Autodesk Inventor part; units mm, degrees
(part 6 of 6)
  arc A2821 (-284.9898, 50) -> (-285.1385, 49.8696) centre (-284.9898, 49.85) ccw
  line L381 (-284.9898, 50) -> (-284.4705, 50)
  arc A2822 (-284.3218, 49.8696) -> (-284.4705, 50) centre (-284.4705, 49.85) ccw
  arc A2823 (-284.3218, 49.8696) -> (-284.2292, 49.5618) centre (-283.3304, 50) ccw
  arc A2824 (-284.2292, 49.5618) -> (-283.7302, 49.25) centre (-283.7304, 49.805) ccw
  arc A2825 (-283.7302, 49.25) -> (-283.2311, 49.5618) centre (-283.73, 49.805) ccw
  arc A2826 (-283.2311, 49.5618) -> (-283.1385, 49.8696) centre (-284.13, 50) ccw
  arc A2827 (-282.9898, 50) -> (-283.1385, 49.8696) centre (-282.9898, 49.85) ccw
  line L382 (-282.9898, 50) -> (-282.4705, 50)
  arc A2828 (-282.3218, 49.8696) -> (-282.4705, 50) centre (-282.4705, 49.85) ccw
  arc A2829 (-282.3218, 49.8696) -> (-282.2292, 49.5618) centre (-281.3304, 50) ccw
  arc A2830 (-282.2292, 49.5618) -> (-281.7302, 49.25) centre (-281.7304, 49.805) ccw
  arc A2831 (-281.7302, 49.25) -> (-281.2311, 49.5618) centre (-281.73, 49.805) ccw
  arc A2832 (-281.2311, 49.5618) -> (-281.1385, 49.8696) centre (-282.13, 50) ccw
  arc A2833 (-280.9898, 50) -> (-281.1385, 49.8696) centre (-280.9898, 49.85) ccw
  line L383 (-280.9898, 50) -> (-280.4705, 50)
  arc A2834 (-280.3218, 49.8696) -> (-280.4705, 50) centre (-280.4705, 49.85) ccw
  arc A2835 (-280.3218, 49.8696) -> (-280.2292, 49.5618) centre (-279.3304, 50) ccw
  arc A2836 (-280.2292, 49.5618) -> (-279.7302, 49.25) centre (-279.7304, 49.805) ccw
  arc A2837 (-279.7302, 49.25) -> (-279.2311, 49.5618) centre (-279.73, 49.805) ccw
  arc A2838 (-279.2311, 49.5618) -> (-279.1385, 49.8696) centre (-280.13, 50) ccw
  arc A2839 (-278.9898, 50) -> (-279.1385, 49.8696) centre (-278.9898, 49.85) ccw
  line L384 (-278.9898, 50) -> (-278.4705, 50)
  arc A2840 (-278.3218, 49.8696) -> (-278.4705, 50) centre (-278.4705, 49.85) ccw
  arc A2841 (-278.3218, 49.8696) -> (-278.2292, 49.5618) centre (-277.3304, 50) ccw
  arc A2842 (-278.2292, 49.5618) -> (-277.7302, 49.25) centre (-277.7304, 49.805) ccw
  arc A2843 (-277.7302, 49.25) -> (-277.2311, 49.5618) centre (-277.73, 49.805) ccw
  arc A2844 (-277.2311, 49.5618) -> (-277.1385, 49.8696) centre (-278.13, 50) ccw
  arc A2845 (-276.9898, 50) -> (-277.1385, 49.8696) centre (-276.9898, 49.85) ccw
  line L385 (-276.9898, 50) -> (-276.4705, 50)
  arc A2846 (-276.3218, 49.8696) -> (-276.4705, 50) centre (-276.4705, 49.85) ccw
  arc A2847 (-276.3218, 49.8696) -> (-276.2292, 49.5618) centre (-275.3304, 50) ccw
  arc A2848 (-276.2292, 49.5618) -> (-275.7302, 49.25) centre (-275.7304, 49.805) ccw
  arc A2849 (-275.7302, 49.25) -> (-275.2311, 49.5618) centre (-275.73, 49.805) ccw
  arc A2850 (-275.2311, 49.5618) -> (-275.1385, 49.8696) centre (-276.13, 50) ccw
  arc A2851 (-274.9898, 50) -> (-275.1385, 49.8696) centre (-274.9898, 49.85) ccw
  line L386 (-274.9898, 50) -> (-274.4705, 50)
  arc A2852 (-274.3218, 49.8696) -> (-274.4705, 50) centre (-274.4705, 49.85) ccw
  arc A2853 (-274.3218, 49.8696) -> (-274.2292, 49.5618) centre (-273.3304, 50) ccw
  arc A2854 (-274.2292, 49.5618) -> (-273.7302, 49.25) centre (-273.7304, 49.805) ccw
  arc A2855 (-273.7302, 49.25) -> (-273.2311, 49.5618) centre (-273.73, 49.805) ccw
  arc A2856 (-273.2311, 49.5618) -> (-273.1385, 49.8696) centre (-274.13, 50) ccw
  arc A2857 (-272.9898, 50) -> (-273.1385, 49.8696) centre (-272.9898, 49.85) ccw
  line L387 (-272.9898, 50) -> (-272.4705, 50)
  arc A2858 (-272.3218, 49.8696) -> (-272.4705, 50) centre (-272.4705, 49.85) ccw
  arc A2859 (-272.3218, 49.8696) -> (-272.2292, 49.5618) centre (-271.3304, 50) ccw
  arc A2860 (-272.2292, 49.5618) -> (-271.7302, 49.25) centre (-271.7304, 49.805) ccw
  arc A2861 (-271.7302, 49.25) -> (-271.2311, 49.5618) centre (-271.73, 49.805) ccw
  arc A2862 (-271.2311, 49.5618) -> (-271.1385, 49.8696) centre (-272.13, 50) ccw
  arc A2863 (-270.9898, 50) -> (-271.1385, 49.8696) centre (-270.9898, 49.85) ccw
  line L388 (-270.9898, 50) -> (-270.4705, 50)
  arc A2864 (-270.3218, 49.8696) -> (-270.4705, 50) centre (-270.4705, 49.85) ccw
  arc A2865 (-270.3218, 49.8696) -> (-270.2292, 49.5618) centre (-269.3304, 50) ccw
  arc A2866 (-270.2292, 49.5618) -> (-269.7302, 49.25) centre (-269.7304, 49.805) ccw
  arc A2867 (-269.7302, 49.25) -> (-269.2311, 49.5618) centre (-269.73, 49.805) ccw
  arc A2868 (-269.2311, 49.5618) -> (-269.1385, 49.8696) centre (-270.13, 50) ccw
  arc A2869 (-268.9898, 50) -> (-269.1385, 49.8696) centre (-268.9898, 49.85) ccw
  line L389 (-268.9898, 50) -> (-268.4705, 50)
  arc A2870 (-268.3218, 49.8696) -> (-268.4705, 50) centre (-268.4705, 49.85) ccw
  arc A2871 (-268.3218, 49.8696) -> (-268.2292, 49.5618) centre (-267.3304, 50) ccw
  arc A2872 (-268.2292, 49.5618) -> (-267.7302, 49.25) centre (-267.7304, 49.805) ccw
  arc A2873 (-267.7302, 49.25) -> (-267.2311, 49.5618) centre (-267.73, 49.805) ccw
  arc A2874 (-267.2311, 49.5618) -> (-267.1385, 49.8696) centre (-268.13, 50) ccw
  arc A2875 (-266.9898, 50) -> (-267.1385, 49.8696) centre (-266.9898, 49.85) ccw
  line L390 (-266.9898, 50) -> (-266.4705, 50)
  arc A2876 (-266.3218, 49.8696) -> (-266.4705, 50) centre (-266.4705, 49.85) ccw
  arc A2877 (-266.3218, 49.8696) -> (-266.2292, 49.5618) centre (-265.3304, 50) ccw
  arc A2878 (-266.2292, 49.5618) -> (-265.7302, 49.25) centre (-265.7304, 49.805) ccw
  arc A2879 (-265.7302, 49.25) -> (-265.2311, 49.5618) centre (-265.73, 49.805) ccw
  arc A2880 (-265.2311, 49.5618) -> (-265.1385, 49.8696) centre (-266.13, 50) ccw
  arc A2881 (-264.9898, 50) -> (-265.1385, 49.8696) centre (-264.9898, 49.85) ccw
  line L391 (-264.9898, 50) -> (-264.4705, 50)
  arc A2882 (-264.3218, 49.8696) -> (-264.4705, 50) centre (-264.4705, 49.85) ccw
  arc A2883 (-264.3218, 49.8696) -> (-264.2292, 49.5618) centre (-263.3304, 50) ccw
  arc A2884 (-264.2292, 49.5618) -> (-263.7302, 49.25) centre (-263.7304, 49.805) ccw
  arc A2885 (-263.7302, 49.25) -> (-263.2311, 49.5618) centre (-263.73, 49.805) ccw
  arc A2886 (-263.2311, 49.5618) -> (-263.1385, 49.8696) centre (-264.13, 50) ccw
  arc A2887 (-262.9898, 50) -> (-263.1385, 49.8696) centre (-262.9898, 49.85) ccw
  line L392 (-262.9898, 50) -> (-262.4705, 50)
  arc A2888 (-262.3218, 49.8696) -> (-262.4705, 50) centre (-262.4705, 49.85) ccw
  arc A2889 (-262.3218, 49.8696) -> (-262.2292, 49.5618) centre (-261.3304, 50) ccw
  arc A2890 (-262.2292, 49.5618) -> (-261.7302, 49.25) centre (-261.7304, 49.805) ccw
  arc A2891 (-261.7302, 49.25) -> (-261.2311, 49.5618) centre (-261.73, 49.805) ccw
  arc A2892 (-261.2311, 49.5618) -> (-261.1385, 49.8696) centre (-262.13, 50) ccw
  arc A2893 (-260.9898, 50) -> (-261.1385, 49.8696) centre (-260.9898, 49.85) ccw
  line L393 (-260.9898, 50) -> (-260.4705, 50)
  arc A2894 (-260.3218, 49.8696) -> (-260.4705, 50) centre (-260.4705, 49.85) ccw
  arc A2895 (-260.3218, 49.8696) -> (-260.2292, 49.5618) centre (-259.3304, 50) ccw
  arc A2896 (-260.2292, 49.5618) -> (-259.7302, 49.25) centre (-259.7304, 49.805) ccw
  arc A2897 (-259.7302, 49.25) -> (-259.2311, 49.5618) centre (-259.73, 49.805) ccw
  arc A2898 (-259.2311, 49.5618) -> (-259.1385, 49.8696) centre (-260.13, 50) ccw
  arc A2899 (-258.9898, 50) -> (-259.1385, 49.8696) centre (-258.9898, 49.85) ccw
  line L394 (-258.9898, 50) -> (-258.4705, 50)
  arc A2900 (-258.3218, 49.8696) -> (-258.4705, 50) centre (-258.4705, 49.85) ccw
  arc A2901 (-258.3218, 49.8696) -> (-258.2292, 49.5618) centre (-257.3304, 50) ccw
  arc A2902 (-258.2292, 49.5618) -> (-257.7302, 49.25) centre (-257.7304, 49.805) ccw
  arc A2903 (-257.7302, 49.25) -> (-257.2311, 49.5618) centre (-257.73, 49.805) ccw
  arc A2904 (-257.2311, 49.5618) -> (-257.1385, 49.8696) centre (-258.13, 50) ccw
  arc A2905 (-256.9898, 50) -> (-257.1385, 49.8696) centre (-256.9898, 49.85) ccw
  line L395 (-256.9898, 50) -> (-256.4705, 50)
  arc A2906 (-256.3218, 49.8696) -> (-256.4705, 50) centre (-256.4705, 49.85) ccw
  arc A2907 (-256.3218, 49.8696) -> (-256.2292, 49.5618) centre (-255.3304, 50) ccw
  arc A2908 (-256.2292, 49.5618) -> (-255.7302, 49.25) centre (-255.7304, 49.805) ccw
  arc A2909 (-255.7302, 49.25) -> (-255.2311, 49.5618) centre (-255.73, 49.805) ccw
  arc A2910 (-255.2311, 49.5618) -> (-255.1385, 49.8696) centre (-256.13, 50) ccw
  arc A2911 (-254.9898, 50) -> (-255.1385, 49.8696) centre (-254.9898, 49.85) ccw
  line L396 (-254.9898, 50) -> (-254.4705, 50)
  arc A2912 (-254.3218, 49.8696) -> (-254.4705, 50) centre (-254.4705, 49.85) ccw
  arc A2913 (-254.3218, 49.8696) -> (-254.2292, 49.5618) centre (-253.3304, 50) ccw
  arc A2914 (-254.2292, 49.5618) -> (-253.7302, 49.25) centre (-253.7304, 49.805) ccw
  arc A2915 (-253.7302, 49.25) -> (-253.2311, 49.5618) centre (-253.73, 49.805) ccw
  arc A2916 (-253.2311, 49.5618) -> (-253.1385, 49.8696) centre (-254.13, 50) ccw
  arc A2917 (-252.9898, 50) -> (-253.1385, 49.8696) centre (-252.9898, 49.85) ccw
  line L397 (-252.9898, 50) -> (-252.4705, 50)
  arc A2918 (-252.3218, 49.8696) -> (-252.4705, 50) centre (-252.4705, 49.85) ccw
  arc A2919 (-252.3218, 49.8696) -> (-252.2292, 49.5618) centre (-251.3304, 50) ccw
  arc A2920 (-252.2292, 49.5618) -> (-251.7302, 49.25) centre (-251.7304, 49.805) ccw
  arc A2921 (-251.7302, 49.25) -> (-251.2311, 49.5618) centre (-251.73, 49.805) ccw
  arc A2922 (-251.2311, 49.5618) -> (-251.1385, 49.8696) centre (-252.13, 50) ccw
  arc A2923 (-250.9898, 50) -> (-251.1385, 49.8696) centre (-250.9898, 49.85) ccw
  line L398 (-250.9898, 50) -> (-250.4705, 50)
  arc A2924 (-250.3218, 49.8696) -> (-250.4705, 50) centre (-250.4705, 49.85) ccw
  arc A2925 (-250.3218, 49.8696) -> (-250.2292, 49.5618) centre (-249.3304, 50) ccw
  arc A2926 (-250.2292, 49.5618) -> (-249.7302, 49.25) centre (-249.7304, 49.805) ccw
  arc A2927 (-249.7302, 49.25) -> (-249.2311, 49.5618) centre (-249.73, 49.805) ccw
  arc A2928 (-249.2311, 49.5618) -> (-249.1385, 49.8696) centre (-250.13, 50) ccw
  arc A2929 (-248.9898, 50) -> (-249.1385, 49.8696) centre (-248.9898, 49.85) ccw
  line L399 (-248.9898, 50) -> (-248.4705, 50)
  arc A2930 (-248.3218, 49.8696) -> (-248.4705, 50) centre (-248.4705, 49.85) ccw
  arc A2931 (-248.3218, 49.8696) -> (-248.2292, 49.5618) centre (-247.3304, 50) ccw
  arc A2932 (-248.2292, 49.5618) -> (-247.7302, 49.25) centre (-247.7304, 49.805) ccw
  arc A2933 (-247.7302, 49.25) -> (-247.2311, 49.5618) centre (-247.73, 49.805) ccw
  arc A2934 (-247.2311, 49.5618) -> (-247.1385, 49.8696) centre (-248.13, 50) ccw
  arc A2935 (-246.9898, 50) -> (-247.1385, 49.8696) centre (-246.9898, 49.85) ccw
  line L400 (-246.9898, 50) -> (-246.4705, 50)
  arc A2936 (-246.3218, 49.8696) -> (-246.4705, 50) centre (-246.4705, 49.85) ccw
  arc A2937 (-246.3218, 49.8696) -> (-246.2292, 49.5618) centre (-245.3304, 50) ccw
  arc A2938 (-246.2292, 49.5618) -> (-245.7302, 49.25) centre (-245.7304, 49.805) ccw
  arc A2939 (-245.7302, 49.25) -> (-245.2311, 49.5618) centre (-245.73, 49.805) ccw
  arc A2940 (-245.2311, 49.5618) -> (-245.1385, 49.8696) centre (-246.13, 50) ccw
  arc A2941 (-244.9898, 50) -> (-245.1385, 49.8696) centre (-244.9898, 49.85) ccw
  line L401 (-244.9898, 50) -> (-244.4705, 50)
  arc A2942 (-244.3218, 49.8696) -> (-244.4705, 50) centre (-244.4705, 49.85) ccw
  arc A2943 (-244.3218, 49.8696) -> (-244.2292, 49.5618) centre (-243.3304, 50) ccw
  arc A2944 (-244.2292, 49.5618) -> (-243.7302, 49.25) centre (-243.7304, 49.805) ccw
  arc A2945 (-243.7302, 49.25) -> (-243.2311, 49.5618) centre (-243.73, 49.805) ccw
  arc A2946 (-243.2311, 49.5618) -> (-243.1385, 49.8696) centre (-244.13, 50) ccw
  arc A2947 (-242.9898, 50) -> (-243.1385, 49.8696) centre (-242.9898, 49.85) ccw
  line L402 (-242.9898, 50) -> (-242.4705, 50)
  arc A2948 (-242.3218, 49.8696) -> (-242.4705, 50) centre (-242.4705, 49.85) ccw
  arc A2949 (-242.3218, 49.8696) -> (-242.2292, 49.5618) centre (-241.3304, 50) ccw
  arc A2950 (-242.2292, 49.5618) -> (-241.7302, 49.25) centre (-241.7304, 49.805) ccw
  arc A2951 (-241.7302, 49.25) -> (-241.2311, 49.5618) centre (-241.73, 49.805) ccw
  arc A2952 (-241.2311, 49.5618) -> (-241.1385, 49.8696) centre (-242.13, 50) ccw
  arc A2953 (-240.9898, 50) -> (-241.1385, 49.8696) centre (-240.9898, 49.85) ccw
  line L403 (-240.9898, 50) -> (-240.4705, 50)
  arc A2954 (-240.3218, 49.8696) -> (-240.4705, 50) centre (-240.4705, 49.85) ccw
  arc A2955 (-240.3218, 49.8696) -> (-240.2292, 49.5618) centre (-239.3304, 50) ccw
  arc A2956 (-240.2292, 49.5618) -> (-239.7302, 49.25) centre (-239.7304, 49.805) ccw
  arc A2957 (-239.7302, 49.25) -> (-239.2311, 49.5618) centre (-239.73, 49.805) ccw
  arc A2958 (-239.2311, 49.5618) -> (-239.1385, 49.8696) centre (-240.13, 50) ccw
  arc A2959 (-238.9898, 50) -> (-239.1385, 49.8696) centre (-238.9898, 49.85) ccw
  line L404 (-238.9898, 50) -> (-238.4705, 50)
  arc A2960 (-238.3218, 49.8696) -> (-238.4705, 50) centre (-238.4705, 49.85) ccw
  arc A2961 (-238.3218, 49.8696) -> (-238.2292, 49.5618) centre (-237.3304, 50) ccw
  arc A2962 (-238.2292, 49.5618) -> (-237.7302, 49.25) centre (-237.7304, 49.805) ccw
  arc A2963 (-237.7302, 49.25) -> (-237.2311, 49.5618) centre (-237.73, 49.805) ccw
  arc A2964 (-237.2311, 49.5618) -> (-237.1385, 49.8696) centre (-238.13, 50) ccw
  arc A2965 (-236.9898, 50) -> (-237.1385, 49.8696) centre (-236.9898, 49.85) ccw
  line L405 (-236.9898, 50) -> (-236.4705, 50)
  arc A2966 (-236.3218, 49.8696) -> (-236.4705, 50) centre (-236.4705, 49.85) ccw
  arc A2967 (-236.3218, 49.8696) -> (-236.2292, 49.5618) centre (-235.3304, 50) ccw
  arc A2968 (-236.2292, 49.5618) -> (-235.7302, 49.25) centre (-235.7304, 49.805) ccw
  arc A2969 (-235.7302, 49.25) -> (-235.2311, 49.5618) centre (-235.73, 49.805) ccw
  arc A2970 (-235.2311, 49.5618) -> (-235.1385, 49.8696) centre (-236.13, 50) ccw
  arc A2971 (-234.9898, 50) -> (-235.1385, 49.8696) centre (-234.9898, 49.85) ccw
  line L406 (-234.9898, 50) -> (-234.4705, 50)
  arc A2972 (-234.3218, 49.8696) -> (-234.4705, 50) centre (-234.4705, 49.85) ccw
  arc A2973 (-234.3218, 49.8696) -> (-234.2292, 49.5618) centre (-233.3304, 50) ccw
  arc A2974 (-234.2292, 49.5618) -> (-233.7302, 49.25) centre (-233.7304, 49.805) ccw
  arc A2975 (-233.7302, 49.25) -> (-233.2311, 49.5618) centre (-233.73, 49.805) ccw
  arc A2976 (-233.2311, 49.5618) -> (-233.1385, 49.8696) centre (-234.13, 50) ccw
  arc A2977 (-232.9898, 50) -> (-233.1385, 49.8696) centre (-232.9898, 49.85) ccw
  line L407 (-232.9898, 50) -> (-232.4705, 50)
  arc A2978 (-232.3218, 49.8696) -> (-232.4705, 50) centre (-232.4705, 49.85) ccw
  arc A2979 (-232.3218, 49.8696) -> (-232.2292, 49.5618) centre (-231.3304, 50) ccw
  arc A2980 (-232.2292, 49.5618) -> (-231.7302, 49.25) centre (-231.7304, 49.805) ccw
  arc A2981 (-231.7302, 49.25) -> (-231.2311, 49.5618) centre (-231.73, 49.805) ccw
  arc A2982 (-231.2311, 49.5618) -> (-231.1385, 49.8696) centre (-232.13, 50) ccw
  arc A2983 (-230.9898, 50) -> (-231.1385, 49.8696) centre (-230.9898, 49.85) ccw
  line L408 (-230.9898, 50) -> (-230.4705, 50)
  arc A2984 (-230.3218, 49.8696) -> (-230.4705, 50) centre (-230.4705, 49.85) ccw
  arc A2985 (-230.3218, 49.8696) -> (-230.2292, 49.5618) centre (-229.3304, 50) ccw
  arc A2986 (-230.2292, 49.5618) -> (-229.7302, 49.25) centre (-229.7304, 49.805) ccw
  arc A2987 (-229.7302, 49.25) -> (-229.2311, 49.5618) centre (-229.73, 49.805) ccw
  arc A2988 (-229.2311, 49.5618) -> (-229.1385, 49.8696) centre (-230.13, 50) ccw
  arc A2989 (-228.9898, 50) -> (-229.1385, 49.8696) centre (-228.9898, 49.85) ccw
  line L409 (-228.9898, 50) -> (-228.4705, 50)
  arc A2990 (-228.3218, 49.8696) -> (-228.4705, 50) centre (-228.4705, 49.85) ccw
  arc A2991 (-228.3218, 49.8696) -> (-228.2292, 49.5618) centre (-227.3304, 50) ccw
  arc A2992 (-228.2292, 49.5618) -> (-227.7302, 49.25) centre (-227.7304, 49.805) ccw
  arc A2993 (-227.7302, 49.25) -> (-227.2311, 49.5618) centre (-227.73, 49.805) ccw
  arc A2994 (-227.2311, 49.5618) -> (-227.1385, 49.8696) centre (-228.13, 50) ccw
  arc A2995 (-226.9898, 50) -> (-227.1385, 49.8696) centre (-226.9898, 49.85) ccw
  line L410 (-226.9898, 50) -> (-226.4705, 50)
  arc A2996 (-226.3218, 49.8696) -> (-226.4705, 50) centre (-226.4705, 49.85) ccw
  arc A2997 (-226.3218, 49.8696) -> (-226.2292, 49.5618) centre (-225.3304, 50) ccw
  arc A2998 (-226.2292, 49.5618) -> (-225.7302, 49.25) centre (-225.7304, 49.805) ccw
  arc A2999 (-225.7302, 49.25) -> (-225.2311, 49.5618) centre (-225.73, 49.805) ccw
  arc A3000 (-225.2311, 49.5618) -> (-225.1385, 49.8696) centre (-226.13, 50) ccw
  arc A3001 (-224.9898, 50) -> (-225.1385, 49.8696) centre (-224.9898, 49.85) ccw
  line L411 (-224.9898, 50) -> (-224.4705, 50)
  arc A3002 (-224.3218, 49.8696) -> (-224.4705, 50) centre (-224.4705, 49.85) ccw
  arc A3003 (-224.3218, 49.8696) -> (-224.2292, 49.5618) centre (-223.3304, 50) ccw
  arc A3004 (-224.2292, 49.5618) -> (-223.7302, 49.25) centre (-223.7304, 49.805) ccw
  arc A3005 (-223.7302, 49.25) -> (-223.2311, 49.5618) centre (-223.73, 49.805) ccw
  arc A3006 (-223.2311, 49.5618) -> (-223.1385, 49.8696) centre (-224.13, 50) ccw
  arc A3007 (-222.9898, 50) -> (-223.1385, 49.8696) centre (-222.9898, 49.85) ccw
  line L412 (-222.9898, 50) -> (-222.4705, 50)
  arc A3008 (-222.3218, 49.8696) -> (-222.4705, 50) centre (-222.4705, 49.85) ccw
  arc A3009 (-222.3218, 49.8696) -> (-222.2292, 49.5618) centre (-221.3304, 50) ccw
  arc A3010 (-222.2292, 49.5618) -> (-221.7302, 49.25) centre (-221.7304, 49.805) ccw
  arc A3011 (-221.7302, 49.25) -> (-221.2311, 49.5618) centre (-221.73, 49.805) ccw
  arc A3012 (-221.2311, 49.5618) -> (-221.1385, 49.8696) centre (-222.13, 50) ccw
  arc A3013 (-220.9898, 50) -> (-221.1385, 49.8696) centre (-220.9898, 49.85) ccw
  line L413 (-220.9898, 50) -> (-220.4705, 50)
  arc A3014 (-220.3218, 49.8696) -> (-220.4705, 50) centre (-220.4705, 49.85) ccw
  arc A3015 (-220.3218, 49.8696) -> (-220.2292, 49.5618) centre (-219.3304, 50) ccw
  arc A3016 (-220.2292, 49.5618) -> (-219.7302, 49.25) centre (-219.7304, 49.805) ccw
  arc A3017 (-219.7302, 49.25) -> (-219.2311, 49.5618) centre (-219.73, 49.805) ccw
  arc A3018 (-219.2311, 49.5618) -> (-219.1385, 49.8696) centre (-220.13, 50) ccw
  arc A3019 (-218.9898, 50) -> (-219.1385, 49.8696) centre (-218.9898, 49.85) ccw
  line L414 (-218.9898, 50) -> (-218.4705, 50)
  arc A3020 (-218.3218, 49.8696) -> (-218.4705, 50) centre (-218.4705, 49.85) ccw
  arc A3021 (-218.3218, 49.8696) -> (-218.2292, 49.5618) centre (-217.3304, 50) ccw
  arc A3022 (-218.2292, 49.5618) -> (-217.7302, 49.25) centre (-217.7304, 49.805) ccw
  arc A3023 (-217.7302, 49.25) -> (-217.2311, 49.5618) centre (-217.73, 49.805) ccw
  arc A3024 (-217.2311, 49.5618) -> (-217.1385, 49.8696) centre (-218.13, 50) ccw
  arc A3025 (-216.9898, 50) -> (-217.1385, 49.8696) centre (-216.9898, 49.85) ccw
  line L415 (-216.9898, 50) -> (-216.4705, 50)
  arc A3026 (-216.3218, 49.8696) -> (-216.4705, 50) centre (-216.4705, 49.85) ccw
  arc A3027 (-216.3218, 49.8696) -> (-216.2292, 49.5618) centre (-215.3304, 50) ccw
  arc A3028 (-216.2292, 49.5618) -> (-215.7302, 49.25) centre (-215.7304, 49.805) ccw
  arc A3029 (-215.7302, 49.25) -> (-215.2311, 49.5618) centre (-215.73, 49.805) ccw
  arc A3030 (-215.2311, 49.5618) -> (-215.1385, 49.8696) centre (-216.13, 50) ccw
  arc A3031 (-214.9898, 50) -> (-215.1385, 49.8696) centre (-214.9898, 49.85) ccw
  line L416 (-214.9898, 50) -> (-214.4705, 50)
  arc A3032 (-214.3218, 49.8696) -> (-214.4705, 50) centre (-214.4705, 49.85) ccw
  arc A3033 (-214.3218, 49.8696) -> (-214.2292, 49.5618) centre (-213.3304, 50) ccw
  arc A3034 (-214.2292, 49.5618) -> (-213.7302, 49.25) centre (-213.7304, 49.805) ccw
  arc A3035 (-213.7302, 49.25) -> (-213.2311, 49.5618) centre (-213.73, 49.805) ccw
  arc A3036 (-213.2311, 49.5618) -> (-213.1385, 49.8696) centre (-214.13, 50) ccw
  arc A3037 (-212.9898, 50) -> (-213.1385, 49.8696) centre (-212.9898, 49.85) ccw
  line L417 (-212.9898, 50) -> (-212.4705, 50)
  arc A3038 (-212.3218, 49.8696) -> (-212.4705, 50) centre (-212.4705, 49.85) ccw
  arc A3039 (-212.3218, 49.8696) -> (-212.2292, 49.5618) centre (-211.3304, 50) ccw
  arc A3040 (-212.2292, 49.5618) -> (-211.7302, 49.25) centre (-211.7304, 49.805) ccw
  arc A3041 (-211.7302, 49.25) -> (-211.2311, 49.5618) centre (-211.73, 49.805) ccw
  arc A3042 (-211.2311, 49.5618) -> (-211.1385, 49.8696) centre (-212.13, 50) ccw
  arc A3043 (-210.9898, 50) -> (-211.1385, 49.8696) centre (-210.9898, 49.85) ccw
  line L418 (-210.9898, 50) -> (-210.4705, 50)
  arc A3044 (-210.3218, 49.8696) -> (-210.4705, 50) centre (-210.4705, 49.85) ccw
  arc A3045 (-210.3218, 49.8696) -> (-210.2292, 49.5618) centre (-209.3304, 50) ccw
  arc A3046 (-210.2292, 49.5618) -> (-209.7302, 49.25) centre (-209.7304, 49.805) ccw
  arc A3047 (-209.7302, 49.25) -> (-209.2311, 49.5618) centre (-209.73, 49.805) ccw
  arc A3048 (-209.2311, 49.5618) -> (-209.1385, 49.8696) centre (-210.13, 50) ccw
  arc A3049 (-208.9898, 50) -> (-209.1385, 49.8696) centre (-208.9898, 49.85) ccw
  line L419 (-208.9898, 50) -> (-208.4709, 50)
  arc A3050 (-208.3222, 49.8696) -> (-208.4709, 50) centre (-208.4709, 49.85) ccw
  arc A3051 (-208.3222, 49.8696) -> (-208.2296, 49.5618) centre (-207.3307, 50) ccw
  arc A3052 (-208.2296, 49.5618) -> (-207.7306, 49.25) centre (-207.7307, 49.805) ccw
  arc A3053 (-207.7306, 49.25) -> (-207.2315, 49.5618) centre (-207.7304, 49.805) ccw
  arc A3054 (-207.2315, 49.5618) -> (-207.1389, 49.8696) centre (-208.1304, 50) ccw
  arc A3055 (-206.9902, 50) -> (-207.1389, 49.8696) centre (-206.9902, 49.85) ccw
  line L420 (-206.9902, 50) -> (-206.4709, 50)
  arc A3056 (-206.3222, 49.8696) -> (-206.4709, 50) centre (-206.4709, 49.85) ccw
  arc A3057 (-206.3222, 49.8696) -> (-206.2296, 49.5618) centre (-205.3307, 50) ccw
  arc A3058 (-206.2296, 49.5618) -> (-205.7306, 49.25) centre (-205.7307, 49.805) ccw
  arc A3059 (-205.7306, 49.25) -> (-205.2315, 49.5618) centre (-205.7304, 49.805) ccw
  arc A3060 (-205.2315, 49.5618) -> (-205.1389, 49.8696) centre (-206.1304, 50) ccw
  arc A3061 (-411.7302, 49.25) -> (-411.7302, 37.03) centre (-411.7302, 43.14) ccw
  line L421 (-411.7302, 49.25) -> (-230.9253, 49.25)
  arc A3062 (-230.9242, 37.03) -> (-230.9253, 49.25) centre (-230.9242, 43.14) ccw
  line L422 (-230.9242, 37.03) -> (-411.7302, 37.03)
  line L423 (-230.9242, 48.62) -> (-411.7302, 48.62)
  arc A3063 (-411.7302, 48.62) -> (-411.7302, 37.66) centre (-411.7302, 43.14) ccw
  line L424 (-411.7302, 37.66) -> (-230.9233, 37.66)
  arc A3064 (-230.9233, 37.66) -> (-230.9242, 48.62) centre (-230.9242, 43.14) ccw
  point P0 (-56.6424, 85.638)
  point P1 (-326.9898, 50)
  dimension "d5" = 180.8049
  dimension "d6" = 0.63
  constraints: 9 point on circle, 8 end point, 4 centre point, 1 horizontal, 3 other
  measures "d5" distance of L421.start L421.end
  measures "d6" distance between parallel lines of L421 L423
extrude "Extrusion1" add sketch "Sketch2" along normal blind 6 contours L421 A3062 L422 A3061
ref_plane "Work Plane3" through (-56.6424, 85.638, -97) normal (0, 0, 1) x (-1, 0, 0)
sketch "Sketch3" plane through (-56.6424, 85.638, -97) normal (0, 0, 1) x (-1, 0, 0)
  arc A0 (-273.7302, 49.25) -> (-273.2311, 49.5618) centre (-273.73, 49.805) ccw
  arc A1 (-274.2292, 49.5618) -> (-273.7302, 49.25) centre (-273.7304, 49.805) ccw
  arc A2 (-274.3218, 49.8696) -> (-274.2292, 49.5618) centre (-273.3304, 50) ccw
  arc A3 (-274.3218, 49.8696) -> (-274.4705, 50) centre (-274.4705, 49.85) ccw
  line L0 (-274.9898, 50) -> (-274.4705, 50)
  arc A4 (-273.2311, 49.5618) -> (-273.1385, 49.8696) centre (-274.13, 50) ccw
  arc A5 (-272.9898, 50) -> (-273.1385, 49.8696) centre (-272.9898, 49.85) ccw
  line L1 (-272.9898, 50) -> (-272.4705, 50)
  arc A6 (-322.6592, 48.4896) -> (-322.8079, 48.62) centre (-322.8079, 48.47) ccw
  arc A7 (-322.6592, 48.4896) -> (-322.5666, 48.1818) centre (-321.6678, 48.62) ccw
  arc A8 (-322.5666, 48.1818) -> (-322.0676, 47.87) centre (-322.0678, 48.425) ccw
  arc A9 (-322.0676, 47.87) -> (-321.5685, 48.1818) centre (-322.0674, 48.425) ccw
  arc A10 (-321.5685, 48.1818) -> (-321.4759, 48.4896) centre (-322.4674, 48.62) ccw
  arc A11 (-321.3272, 48.62) -> (-321.4759, 48.4896) centre (-321.3272, 48.47) ccw
  arc A12 (-230.9242, 37.03) -> (-230.9253, 49.25) centre (-230.9242, 43.14) ccw
  line L2 (-230.9253, 49.25) -> (-411.7302, 49.25)
  arc A13 (-411.7302, 49.25) -> (-411.7302, 37.03) centre (-411.7302, 43.14) ccw
  line L3 (-411.7302, 37.03) -> (-230.9242, 37.03)
  arc A14 (-230.9233, 37.66) -> (-230.9242, 48.62) centre (-230.9242, 43.14) ccw
  line L4 (-230.9233, 37.66) -> (-411.7302, 37.66)
  arc A15 (-411.7302, 48.62) -> (-411.7302, 37.66) centre (-411.7302, 43.14) ccw
  line L5 (-411.7302, 48.62) -> (-230.9242, 48.62)
  point P0 (-56.6424, 85.638)
  point P1 (-321.3272, 48.62)
  point P2 (-322.8079, 48.62)
  constraints: 12 point on circle, 6 centre point
extrude "Extrusion2" add sketch "Sketch3" along normal blind 6 contours A6 L5 A11 A10 A9 A8 A7
body "Solid1"
